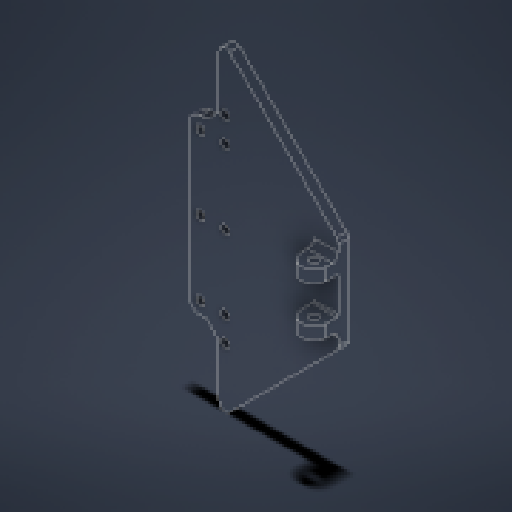
# Autodesk Inventor part: wedge
Saved by Autodesk Inventor 2025.2 (Build 292293000, 293)
## iProperties
Created: 2025-12-02
Part Number: wedge
Material: Generic
Document SubType Name: Modeling
Designer: cloudy
Density: 1 g/cm^3
Appearance: Default
Author: cloudy
Autodesk Inventor part; units mm, degrees
ref_plane "YZ Plane" through (0, 0, 0) normal (1, 0, 0) x (0, 1, 0)
ref_plane "XZ Plane" through (0, 0, 0) normal (0, 1, 0) x (-1, 0, 0)
ref_plane "XY Plane" through (0, 0, 0) normal (0, 0, 1) x (1, 0, 0)
sketch "Sketch1" plane through (0, 0, 0) normal (0, 0, 1) x (1, 0, 0)
  line L0 (88.9, 0) -> (-12.7, 101.6)
  line L1 (-12.7, 101.6) -> (-12.7, -101.6)
  line L2 (-12.7, -101.6) -> (88.9, 0)
  line L3 (-12.7, 0) -> (88.9, 0)
  line L4 (64.73, 183.898) -> (-316.27, 183.898)
  line L5 (-316.27, 183.898) -> (-316.27, -183.898)
  line L6 (-316.27, -183.898) -> (64.73, -183.898)
  line L7 (64.73, -183.898) -> (64.73, 183.898)
  line L8 (64.73, 183.898) -> (-316.27, -183.898) construction
  line L9 (-316.27, 183.898) -> (64.73, -183.898) construction
  circle A0 centre (6.35, 38.1) radius 2.1844 projected
  circle A1 centre (-6.35, 38.1) radius 2.1844 projected
  circle A2 centre (-6.35, -38.1) radius 2.1844 projected
  circle A3 centre (6.35, -38.1) radius 2.1844 projected
  circle A4 centre (6.35, 0) radius 2.1844 projected
  circle A5 centre (6.35, 88.9) radius 2.1844 projected
  circle A6 centre (6.35, 50.8) radius 2.1844 projected
  circle A7 centre (6.35, -50.8) radius 2.1844 projected
  circle A8 centre (-6.35, 0) radius 2.1844 projected
  circle A9 centre (-6.35, 38.1) radius 6.35
  circle A10 centre (-6.35, -38.1) radius 6.35
  line L10 (3.175, -85.725) -> (3.175, -44.45)
  line L11 (3.175, -44.45) -> (-11.204, -44.45)
  line L12 (-10.742, 44.45) -> (3.175, 44.45)
  line L13 (3.175, 44.45) -> (3.175, 85.725)
  point P0 (0, 0)
  point P1 (-125.77, 0)
  point P2 (64.73, 24.17)
  point P3 (-6.35, 44.45)
  point P4 (-12.7, 38.1)
  point P5 (-12.7, -38.1)
  point P6 (-6.35, -44.45)
  point P7 (64.73, -24.17)
  dimension "d0" = 101.6
  dimension "d2" = 381
  dimension "d4" = 12.7
  dimension "d5" = 12.7
  dimension "d6" = 3.175
  dimension "d7" = 3.175
  constraints: 28 end point, 4 vertical, 3 horizontal, 3 midpoint, 3 perpendicular, 3 point on line, 3 tangent, 2 centre point, 2 coincident, 2 parallel
  measures "d0" distance of L3.start L0.start
  measures "d2" distance of L5.end L6.end
  measures "d4" diameter of A9
  measures "d5" diameter of A10
  measures "d6" distance from line of A7.centre L10
  measures "d7" distance from line of L13 A6.centre
extrude "Extrusion1" add sketch "Sketch1" along normal blind 5.08 contours L0 L7 L3 A4 A8 L1 A9 L12 L13 | A9 | L7 L2 L10 L11 A10 L1 L3 A8 A4 | A10
chamfer "Chamfer1" distance 6.35 angle 45 2 edges at (3.175, 44.45, 2.54) (3.175, -44.45, 2.54)
fillet "Fillet1" radius 3.175 4 edges at (3.175, 85.725, 2.54) (3.175, -85.725, 2.54) (64.73, 24.17, 2.54) (64.73, -24.17, 2.54)
sketch "Sketch2" plane through (0, 0, 5.08) normal (0, 0, 1) x (1, 0, 0)
  circle A0 centre (58.38, 0) radius 2.1844
  line L0 (58.38, 0) -> (0, 0) construction
  circle A1 centre (58.38, 12.7) radius 2.1844
  circle A2 centre (58.38, -12.7) radius 2.1844
  line L1 (58.38, 0) -> (58.38, -12.7) construction
  line L2 (64.73, -22.8548) -> (64.73, 22.8548) construction
  line L3 (52.03, -15.875) -> (64.73, -15.875)
  line L4 (64.73, -15.875) -> (64.73, -9.525)
  line L5 (64.73, -9.525) -> (52.03, -9.525)
  line L6 (52.03, -9.525) -> (52.03, -15.875)
  line L7 (52.03, -15.875) -> (64.73, -9.525) construction
  line L8 (64.73, -15.875) -> (52.03, -9.525) construction
  line L9 (52.03, 15.875) -> (64.73, 15.875)
  line L10 (64.73, 15.875) -> (64.73, 9.525)
  line L11 (64.73, 9.525) -> (52.03, 9.525)
  line L12 (52.03, 9.525) -> (52.03, 15.875)
  line L13 (52.03, 15.875) -> (64.73, 9.525) construction
  line L14 (64.73, 15.875) -> (52.03, 9.525) construction
  dimension "d14" = 4.3688
  dimension "d15" = 12.7
  dimension "d16" = 6.35
  dimension "d17" = 12.7
  dimension "d18" = 6.35
  dimension "d19" = 12.7
  dimension "d20" = 6.35
  constraints: 28 end point, 4 midpoint, 4 parallel, 3 centre point, 3 horizontal, 2 perpendicular, 1 equal radius, 1 vertical, 1 other
  measures "d14" diameter of A0
  measures "d15" distance of L0.start L1.end
  measures "d16" distance from line of L2 L0.start
  measures "d17" distance of L5.end L4.end
  measures "d18" distance of L4.end L3.end
  measures "d19" distance of L10.end L11.end
  measures "d20" distance of L9.end L10.end
extrude "Extrusion2" add sketch "Sketch2" along normal blind 12.7 contours A1 | A2 | L6 L5 L4 L3 | L9 L10 L11 L12
fillet "Fillet2" radius 3.175 2 edges at (58.38, -15.875, 5.08) (58.38, 15.875, 5.08)
fillet "Fillet3" radius 6.35 4 edges at (64.73, -12.7, 17.78) (64.73, 12.7, 17.78) (52.03, 12.7, 17.78) (52.03, -12.7, 17.78)
sketch "Sketch3" plane through (52.03, -15.875, 8.255) normal (0, -1, 0) x (1, 0, 0)
  arc A0 (12.7, 3.175) -> (0, 3.175) centre (6.35, 3.175) ccw projected
  circle A1 centre (6.35, 3.175) radius 2.1844
  point P0 (-52.03, -8.255)
  dimension "d28" = 4.3688
  constraints: 1 centre point, 1 coincident
  measures "d28" diameter of A1
extrude "Extrusion3" cut sketch "Sketch3" against normal through all
chamfer "Chamfer3" distance 0.7937 angle 45 2 edges at (58.38, -9.525, 5.08) (58.38, 9.525, 5.08)
body "Solid1"
